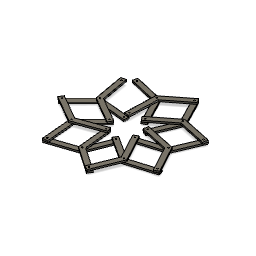
Backgeound design Version 2 v2 (Autodesk Fusion 360 design; units mm, degrees)
Autodesk Fusion 360 part; units mm, degrees
sketch "Sketch1" plane through (0, 0, 0) normal (0, 1, 0) x (1, 0, 0)
  line L0 (-24.4385, -26.1269) -> (-113.0001, -26.1269)
  line L1 (-113.0001, -26.1269) -> (-113.0001, -41.1269)
  line L2 (-113.0001, -41.1269) -> (-17.4439, -41.1269)
  circle A0 centre (-21.0001, -33.6269) radius 2
  circle A1 centre (-105.0001, -33.6269) radius 2
  line L3 (-113.0001, -41.1269) -> (-17.4439, -41.1269)
  circle A2 centre (-21.0001, -33.6269) radius 2
  line L4 (-24.4385, -26.1269) -> (-113.0001, -26.1269)
  line L5 (-17.4439, -41.1269) -> (43.9209, 32.0048)
  line L6 (32.4302, 41.6466) -> (-24.4385, -26.1269)
  line L7 (-17.4439, -41.1269) -> (43.9209, 32.0048)
  circle A3 centre (33.0333, 30.6973) radius 2
  line L8 (32.4302, 41.6466) -> (-24.4385, -26.1269)
  circle A4 centre (-20.9609, -33.6504) radius 2
  line L9 (43.9209, 32.0048) -> (32.4302, 41.6466)
  circle A5 centre (-20.9609, -33.6504) radius 2
  dimension "d6" = 15
  dimension "d7" = 4
  dimension "d8" = 4
  dimension "d10" = 8
  dimension "d11" = 7.5
  dimension "d12" = 7.5
  dimension "d14" = 15
  dimension "d15" = 4
  dimension "d17" = 7.5
  dimension "d19" = 15
  dimension "d20" = 4
  dimension "d21" = 4
  dimension "d23" = 8
  dimension "d24" = 7.5
  dimension "d25" = 7.5
  dimension "d27" = 15
  dimension "d28" = 4
  dimension "d30" = 7.5
  constraint horizontal L0
  constraint vertical L1
  constraint horizontal L2
  constraint horizontal L4
  constraint horizontal L3
  measures "d6" distance of L0.end L1.end
  measures "d7" diameter of A1
  measures "d8" diameter of A0
  measures "d10" distance of L1 A1.centre
  measures "d11" distance of L0 A1.centre
  measures "d12" distance of L0 A0.centre
  measures "d14" distance of L1.end L0.end
  measures "d15" diameter of A2
  measures "d17" distance of A0.centre L4
  measures "d19" distance of L6.start L5.end
  measures "d20" diameter of A3
  measures "d21" diameter of A4
  measures "d23" distance of A3.centre L9
  measures "d24" distance of A3.centre L5
  measures "d25" distance of A4.centre L5
  measures "d27" distance of L6.start L5.end
  measures "d28" diameter of A5
  measures "d30" distance of A4.centre L7
extrude "Extrude1" add sketch "Sketch1" along normal blind 5 makes body 1
copy_body "CopyPasteBodies1" bodies 1 makes body 2
move_body "Move1" bodies 2 to x (1, 0, 0) y (0, 1, 0) z (0, 0, 1) at (-27.5951, 0, -46.2286)
copy_body "CopyPasteBodies2" bodies 1 makes body 3
move_body "Move2" bodies 3 to x (1, 0, 0) y (0, 1, 0) z (0, 0, 1) at (-38.6924, 0, -78.4305)
copy_body "CopyPasteBodies3" bodies 1 makes body 4
move_body "Move3" bodies 4 to x (1, 0, 0) y (0, 1, 0) z (0, 0, 1) at (14.2918, 0, 33.1151)
copy_body "CopyPasteBodies4" bodies 1 makes body 5
move_body "Move4" bodies 5 to x (1, 0, 0) y (0, 1, 0) z (0, 0, 1) at (26.4921, 0, 57.8643)
copy_body "CopyPasteBodies5" bodies 1 makes body 6
move_body "Move5" bodies 6 to x (1, 0, 0) y (0, 1, 0) z (0, 0, 1) at (-11.5031, 0, -24.052)
copy_body "CopyPasteBodies6" bodies 1 makes body 7
move_body "Move6" bodies 7 to x (1, 0, 0) y (0, 1, 0) z (0, 0, 1) at (-50.1955, 0, -101.7854)
copy_body "CopyPasteBodies7" bodies 1 makes body 8
move_body "Move7" bodies 8 to x (1, 0, 0) y (0, 1, 0) z (0, 0, 1) at (-63.4416, 0, -123.746)
copy_body "Body->Comp1" bodies 1 removing the originals makes body 9 in component "Component"
copy_body "Body->Comp2" bodies 2 removing the originals makes body 10 in component "Component'"
copy_body "Body->Comp3" bodies 3 removing the originals makes body 11 in component "Component''"
copy_body "Body->Comp4" bodies 4 removing the originals makes body 12 in component "Component'''"
copy_body "Body->Comp5" bodies 5 removing the originals makes body 13 in component "Component''''"
copy_body "Body->Comp6" bodies 6 removing the originals makes body 14 in component "Component'''''"
copy_body "Body->Comp7" bodies 7 removing the originals makes body 15 in component "Component''''''"
copy_body "Body->Comp8" bodies 8 removing the originals makes body 16 in component "Component'''''''"
move_body "Move1'" bodies 9 to x (1, 0, 0) y (0, 1, 0) z (0, 0, 1) at (-14.0048, 0, -35.5507) in component "Component"
move_body "Move1''" bodies 11 to x (1, 0, 0) y (0, 1, 0) z (0, 0, 1) at (-14.0048, 0, -35.5507) in component "Component''"
move_body "Move1'''" bodies 15 to x (1, 0, 0) y (0, 1, 0) z (0, 0, 1) at (-14.0048, 0, -35.5507) in component "Component''''''"
move_body "Move1''''" bodies 16 to x (1, 0, 0) y (0, 1, 0) z (0, 0, 1) at (-14.0048, 0, -35.5507) in component "Component'''''''"
move_body "Move1'''''" bodies 10 to x (1, 0, 0) y (0, 1, 0) z (0, 0, 1) at (-14.0048, 0, -35.5507) in component "Component'"
move_body "Move1''''''" bodies 14 to x (1, 0, 0) y (0, 1, 0) z (0, 0, 1) at (-14.0048, 0, -35.5507) in component "Component'''''"
move_body "Move1'''''''" bodies 13 to x (0.087156, 0, 0.996195) y (0, 1, 0) z (-0.996195, 0, 0.087156) at (32.0186, 0, 194.3019) in component "Component''''"
copy_body "CopyPasteBodies8" bodies 1
copy_body "CopyPasteBodies9" bodies 10 makes body 17
move_body "Move8" bodies 17 to x (1, 0, 0) y (0, 1, 0) z (0, 0, 1) at (14.2402, 0, 30.5778)
copy_body "CopyPasteBodies10" bodies 10 makes body 18
move_body "Move9" bodies 18 to x (1, 0, 0) y (0, 1, 0) z (0, 0, 1) at (-47.5002, 0, -106.0752)
copy_body "CopyPasteBodies11" bodies 10 makes body 19
move_body "Move10" bodies 19 to x (1, 0, 0) y (0, 1, 0) z (0, 0, 1) at (-60.7143, 0, -133.2114)
copy_body "CopyPasteBodies12" bodies 10 makes body 20
move_body "Move11" bodies 20 to x (1, 0, 0) y (0, 1, 0) z (0, 0, 1) at (-75.5449, 0, -160.0938)
copy_body "CopyPasteBodies13" bodies 10 makes body 21
move_body "Move12" bodies 21 to x (1, 0, 0) y (0, 1, 0) z (0, 0, 1) at (-88.6465, 0, -189.0004)
copy_body "CopyPasteBodies14" bodies 10 makes body 22
move_body "Move13" bodies 22 to x (1, 0, 0) y (0, 1, 0) z (0, 0, 1) at (-100.1033, 0, -213.0045)
move_body "Move14" bodies 17 to x (1, 0, 0) y (0, 1, 0) z (0, 0, 1) at (-128.3026, 0, -267.3884)
move_body "Move2'" bodies 10 to x (1, 0, 0) y (0, 1, 0) z (0, 0, 1) at (-128.3026, 0, -267.3884) in component "Component'"
copy_body "Body->Comp9" bodies 17 removing the originals makes body 23 in component "Component''''''''"
copy_body "Body->Comp10" bodies 18 removing the originals makes body 24 in component "Component'''''''''"
copy_body "Body->Comp12" bodies 20 removing the originals makes body 25 in component "Component''''''''''"
copy_body "Body->Comp13" bodies 21 removing the originals makes body 26 in component "Component'''''''''''"
copy_body "Body->Comp14" bodies 22 removing the originals makes body 27 in component "Component''''''''''''"
copy_body "Body->Comp15" bodies 19 removing the originals makes body 28 in component "Component'''''''''''''"
component "Component" placed x (0.917923, 0, -0.396758) y (0, 1, 0) z (0.396758, 0, 0.917923) at (-68.0832, -5, 115.5054)
component "Component'" placed x (-0.68334, 0, -0.730101) y (0, 1, 0) z (0.730101, 0, -0.68334) at (-64.1686, 0, -497.1675)
component "Component''" placed x (0.25199, 0, 0.96773) y (0, 1, 0) z (-0.96773, 0, 0.25199) at (-302.7179, 5, 64.5143)
component "Component'''" placed x (0.903217, 0, 0.429185) y (0, 1, 0) z (-0.429185, 0, 0.903217) at (-173.5927, 5, 25.1183)
component "Component''''" placed x (0.957296, 0, -0.289108) y (0, 1, 0) z (0.289108, 0, 0.957296) at (-104.6045, 0, -90.2269)
component "Component'''''" placed x (-0.483427, 0, 0.875385) y (0, 1, 0) z (-0.875385, 0, -0.483427) at (-253.4932, 0, 110.7147)
component "Component''''''" placed x (-0.981294, 0, 0.192518) y (0, 1, 0) z (-0.192518, 0, -0.981294) at (-347.1, 0, -112.4198)
component "Component'''''''" placed x (0.957061, 0, 0.289885) y (0, 1, 0) z (-0.289885, 0, 0.957061) at (61.2818, 0, 220.3073)
component "Component''''''''" placed x (-0.729675, 0, 0.683794) y (0, 1, 0) z (-0.683794, 0, -0.729675) at (-487.856, 5, -229.2977)
component "Component'''''''''" placed x (0.290287, 0, -0.95694) y (0, 1, 0) z (0.95694, 0, 0.290287) at (183.0395, 5, 10.9066)
component "Component''''''''''" placed x (0.837337, 0, -0.546686) y (0, 1, 0) z (0.546686, 0, 0.837337) at (257.4786, 0, 54.0452)
component "Component'''''''''''" placed x (-0.546321, 0, -0.837576) y (0, 1, 0) z (0.837576, 0, -0.546321) at (143.9653, 5, -301.0017)
component "Component''''''''''''" placed x (0.119514, 0, -0.992832) y (0, 1, 0) z (0.992832, 0, 0.119514) at (233.3348, 0, -268.598)
component "Component'''''''''''''" placed x (-0.992832, 0, -0.119514) y (0, 1, 0) z (0.119514, 0, -0.992832) at (-146.1145, 5, -333.0467)
equation "lenth = 100 mm"
equation "width = 15 mm"
equation "boltM4 = 4 mm"
equation "Thickness = 5 mm"
equation "d6 = width"
equation "d7 = boltM4"
equation "d8 = boltM4"
equation "d14 = width"
equation "d15 = boltM4"
equation "d19 = width"
equation "d20 = boltM4"
equation "d21 = boltM4"
equation "d27 = width"
equation "d28 = boltM4"
equation "d31 = Thickness"
